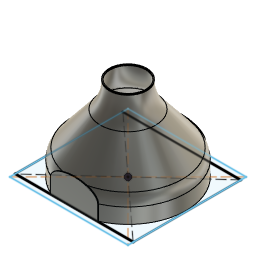
2023_05_26_AirFlow V2 Heavy Cuver with Weight Circle v5 (Autodesk Fusion 360 design; units mm, degrees)
Autodesk Fusion 360 part; units mm, degrees
sketch "Sketch2" plane through (0, 0, 0) normal (0, 0, 1) x (1, 0, 0)
  circle A0 centre (0, 0) radius 111.5
  line L0 (-115, -115) -> (115, -115)
  line L1 (115, -115) -> (115, 115)
  line L2 (115, 115) -> (-115, 115)
  line L3 (-115, 115) -> (-115, -115)
  line L4 (-115, -115) -> (115, 115) construction
  line L5 (115, -115) -> (-115, 115) construction
  dimension "d9" = 223
  dimension "d10" = 230
  dimension "d11" = 230
  constraint coincident A0.centre origin
  constraint horizontal L0
  constraint perpendicular L0 L1
  constraint parallel L0 L2
  constraint parallel L1 L3
  constraint coincident L4 A0.centre
  constraint coincident L5 A0.centre
  measures "d9" diameter of A0
  measures "d10" distance of L1.end L2.end
  measures "d11" distance of L0.end L1.end
sketch "Sketch1" plane through (0, 0, 0) normal (1, 0, 0) x (0, 1, 0)
  line L0 (0, 0) -> (-111.5, 0) construction
  line L1 (-111.5, 0) -> (-111.5, 29.3764)
  line L2 (0, 135) -> (-34.5705, 135) construction
  line L3 (-104.8144, 48.2561) -> (-52.3988, 112.9839)
  line L4 (-111.5, 40) -> (55.6546, 40) construction
  line L5 (-34.5705, 163.3295) -> (-34.5705, 165)
  line L6 (-113.3, 0) -> (-111.5, 0)
  line L7 (-36.3705, 165) -> (-34.5705, 165)
  arc A0 (-104.8144, 48.2561) -> (-111.5, 29.3764) centre (-81.5, 29.3764) ccw
  arc A1 (-52.3988, 112.9839) -> (-34.5705, 163.3295) centre (-114.5705, 163.3295) ccw
  line L8 (-113.3, 0) -> (-113.3, 29.3764)
  arc A2 (-106.2132, 49.3888) -> (-113.3, 29.3764) centre (-81.5, 29.3764) ccw
  line L9 (-106.2132, 49.3888) -> (-53.7977, 114.1166)
  arc A3 (-53.7977, 114.1166) -> (-36.3705, 163.3295) centre (-114.5705, 163.3295) ccw
  line L10 (-36.3705, 163.3295) -> (-36.3705, 165)
  line L11 (-61.8195, 105.9471) -> (-70.3491, 95.9248)
  line L12 (-70.3491, 95.9248) -> (-73.6764, 95.9248)
  line L13 (-73.6764, 95.9248) -> (-83.351, 105.9471)
  line L14 (-83.351, 105.9471) -> (-83.351, 118.2647)
  line L15 (-63.3425, 107.2434) -> (-71.2733, 97.9248)
  line L16 (-71.2733, 97.9248) -> (-72.8272, 97.9248)
  line L17 (-72.8272, 97.9248) -> (-81.351, 106.755)
  line L18 (-81.351, 106.755) -> (-81.351, 118.2647)
  line L19 (-61.8195, 105.9471) -> (-63.3425, 107.2434)
  line L20 (-81.351, 118.2647) -> (-83.351, 118.2647)
  dimension "d1" = 111.5
  dimension "d2" = 40
  dimension "d4" = 51
  dimension "d5" = 30
  dimension "d6" = -1.8
  dimension "d7" = 30
  dimension "d8" = 80
  dimension "d13" = 2
  constraint coincident L0.start origin
  constraint horizontal L0
  constraint perpendicular L0 L1
  constraint horizontal L2
  constraint horizontal L4
  constraint perpendicular L2 L5
  constraint perpendicular L1 L6
  constraint perpendicular L5 L7
  constraint coincident L4.start L1
  constraint coincident L4.start L3
  constraint tangent L1 A0
  constraint tangent L3 A0
  constraint coincident L3 L2.end
  constraint coincident L2.end L5
  constraint tangent L3 A1
  constraint tangent L5 A1
  constraint horizontal L12
  constraint vertical L14
  constraint perpendicular L14 L20
  measures "d1" distance of L0.start L0.end
  measures "d2" distance of L0.end L4.start
  measures "d4" angle of L3 L4
  measures "d5" distance of L2.end L5.end
  measures "d7" radius of A0
  measures "d8" radius of A1
revolve "Revolve1" add sketch "Sketch1" angle 360 about axis through (0, 0, 1.75) along (0, 0, 1) contours L1 L3 L5 L6 L7 A0 A1 L8 A2 L9 A3 L10 makes body 1
sketch "Sketch3" plane through (0, 0, 0) normal (0, 0, 1) x (1, 0, 0)
revolve "Revolve2" add sketch "Sketch1" angle 360 about axis through (0, 0, 1.75) along (0, 0, 1) separate body contours L11 L12 L13 L14 L15 L16 L17 L18 L19 L20 makes body 2
move_body "Move1" bodies 2 to x (1, 0, 0) y (0, 1, 0) z (0, 0, 1) at (0, 0, -95.9248)
copy_body "CopyPasteBodies1" bodies 1 makes body 3
move_body "Move2" bodies 3 to x (1, 0, 0) y (0, 1, 0) z (0, 0, 1) at (0, 0, 0)
sketch "Sketch4" plane through (0, 0, 0) normal (0, 0, 1) x (1, 0, 0)
  line L0 (115, 105) -> (-115, 105)
  line L1 (-115, 105) -> (-115, -105)
  line L2 (-115, -105) -> (115, -105)
  line L3 (115, -105) -> (115, 105)
  line L4 (115, 105) -> (-115, -105) construction
  line L5 (-115, 105) -> (115, -105) construction
  line L6 (-115, 115) -> (-115, -115)
  line L7 (-115, -115) -> (115, -115)
  line L8 (115, -115) -> (115, 115)
  line L9 (115, 115) -> (-115, -115) construction
  line L10 (-115, 115) -> (115, -115) construction
  line L11 (-115, 105) -> (115, 105)
  line L12 (115, 105) -> (115, 103.5)
  line L13 (115, 103.5) -> (-115, 103.5)
  line L14 (-115, 103.5) -> (-115, 105)
  line L15 (-115, -105) -> (115, -105)
  line L16 (115, -105) -> (115, -103.5)
  line L17 (115, -103.5) -> (-115, -103.5)
  line L18 (-115, -103.5) -> (-115, -105)
  line L19 (115, 115) -> (-115, 115)
  dimension "d15" = 230
  dimension "d16" = 210
  dimension "d17" = 230
  dimension "d18" = 230
  dimension "d21" = 1.5
  dimension "d22" = 1.5
  constraint horizontal L0
  constraint perpendicular L0 L1
  constraint parallel L0 L2
  constraint parallel L1 L3
  constraint coincident L4 origin
  constraint coincident L5 origin
  constraint parallel L6 L8
  constraint coincident L9 origin
  constraint coincident L10 origin
  constraint horizontal L11
  constraint vertical L12
  constraint horizontal L13
  constraint vertical L14
  constraint horizontal L15
  constraint vertical L16
  constraint horizontal L17
  constraint vertical L18
  constraint perpendicular L6 L19
  measures "d15" distance of L1.end L2.end
  measures "d16" distance of L0.end L1.end
  measures "d17" distance of L6.end L7.end
  measures "d18" distance of L6.start L6.end
  measures "d21" distance of L0.end L13.end
  measures "d22" distance of L1.end L17.end
extrude "Extrude1" cut sketch "Sketch4" along normal blind 140 contours L0 L6 L8 L11 L19 | L2 L6 L7 L8 L15 bodies 3
extrude "Extrude2" add sketch "Sketch4" along normal blind 60 contours L0 L1 L3 L6 L8 L11 L12 L13 L14 | L1 L2 L3 L6 L8 L15 L16 L17 L18 bodies 3
extrude "Extrude3" cut 1 faces at (92.0313, -103.5, 29.7921) along direction (0, -1, 0) blind 40 on bodies 3 bodies 3
extrude "Extrude4" cut 1 faces at (92.0313, 103.5, 29.7921) along direction (0, 1, 0) blind 20 on bodies 3 bodies 3
fillet "Fillet1" [suppressed]
move_body "Move3" [suppressed]
sketch "Sketch5" plane through (0, 0, 0) normal (0, 1, 0) x (1, 0, 0)
  line L0 (18.2359, -128.4928) -> (-18.2359, -128.4928)
  line L1 (-18.2359, -119.5072) -> (-18.2359, -116.5072)
  line L2 (18.2359, -116.5072) -> (18.2359, -119.5072)
  line L3 (18.2359, -128.4928) -> (-18.2359, -111.5072) construction
  line L4 (-2.5773, -116.5072) -> (-2.5773, -120)
  arc A0 (-2.5773, -120) -> (2.5773, -120) centre (0, -120) ccw
  line L5 (2.5773, -120) -> (2.5773, -116.5072)
  line L6 (0, -103.0145) -> (0, -120) construction
  line L7 (-13.2359, -111.5072) -> (-7.5773, -111.5072)
  line L8 (7.5773, -111.5072) -> (13.2359, -111.5072)
  arc A1 (-2.5773, -116.5072) -> (-7.5773, -111.5072) centre (-7.5773, -116.5072) ccw
  arc A2 (7.5773, -111.5072) -> (2.5773, -116.5072) centre (7.5773, -116.5072) ccw
  arc A3 (18.2359, -116.5072) -> (13.2359, -111.5072) centre (13.2359, -116.5072) ccw
  arc A4 (-13.2359, -111.5072) -> (-18.2359, -116.5072) centre (-13.2359, -116.5072) ccw
  line L9 (-21.7601, -121.5072) -> (-21.7601, -123.5633)
  line L10 (-21.7601, -123.5633) -> (21.4175, -123.5633)
  line L11 (21.4175, -123.5633) -> (21.4175, -121.5072)
  line L12 (21.4175, -121.5072) -> (-21.7601, -123.5633) construction
  line L13 (-21.7601, -121.5072) -> (21.4175, -123.5633) construction
  line L14 (-18.2359, -128.4928) -> (-4.9547, -122.3075) construction
  line L15 (-3.2364, -121.5072) -> (18.2359, -111.5072) construction
  line L16 (21.4175, -121.5072) -> (20.2359, -121.5072)
  line L17 (-20.2359, -121.5072) -> (-21.7601, -121.5072)
  arc A5 (-20.2359, -121.5072) -> (-18.2359, -119.5072) centre (-20.2359, -119.5072) ccw
  arc A6 (18.2359, -119.5072) -> (20.2359, -121.5072) centre (20.2359, -119.5072) ccw
  point P0 (0, -120)
  point P1 (-0.1713, -122.5353)
  dimension "d34" = 5
  dimension "d53" = 2
  dimension "d54" = 2
  dimension "d55" = 3
  constraint horizontal L0
  constraint perpendicular L0 L1
  constraint parallel L0 L7
  constraint parallel L1 L2
  constraint coincident L3 P0
  constraint coincident P0 L14
  constraint tangent L4 A0
  constraint tangent A0 L5
  constraint parallel L4 L5
  constraint coincident P0 A0.centre
  constraint perpendicular L6 L7
  constraint collinear L7 L8
  constraint tangent L4 A1
  constraint tangent L7 A1
  constraint tangent L5 A2
  constraint tangent L8 A2
  constraint equal A1 A2
  constraint coincident L15.end L2
  constraint coincident L15.end L8
  constraint tangent L2 A3
  constraint tangent L8 A3
  constraint equal A1 A3
  constraint coincident L3.end L7
  constraint coincident L3.end L1
  constraint tangent L7 A4
  constraint tangent L1 A4
  constraint equal A1 A4
  constraint horizontal L16
  constraint perpendicular L9 L16
  constraint parallel L10 L16
  constraint parallel L9 L11
  constraint coincident L12 P1
  constraint coincident L13 P1
  constraint coincident L13 L14.end
  constraint coincident L15.start L16
  constraint collinear L14 L15
  constraint collinear L16 L17
  constraint tangent L17 A5
  constraint tangent L1 A5
  constraint tangent L16 A6
  constraint tangent L2 A6
  measures "d34" radius of A1
  measures "d53" radius of A5
  measures "d54" radius of A6
  measures "d55" distance of L1.end L1.start
extrude "Extrude5" [suppressed]
move_body "Move4" [suppressed]
move_body "Move5" [suppressed]
move_body "Move6" [suppressed]
move_body "Move8" [suppressed]
move_body "Move10" [suppressed]
move_body "Move11" [suppressed]
move_body "Move12" [suppressed]
move_body "Move13" [suppressed]
move_body "Move14" [suppressed]
extrude "Extrude7" [suppressed]
pattern_circular "C-Pattern2" [suppressed]
copy_body "CopyPasteBodies2" [suppressed]
move_body "Move7" [suppressed]
extrude "Extrude6" [suppressed]
combine "Combine2" [suppressed]
move_body "Move9" [suppressed]
pattern_circular "C-Pattern1" [suppressed]
combine "Combine1" [suppressed]
delete_body "RemoveBody2" bodies 4
move_body "Move15" [suppressed]
hidden bodies 1
equation "d1 = 223 mm / 2"
equation "d70 = micron"
named bodies: "Top Weight Circle", "EnderVersion", "Top Weight Circle (1)"
